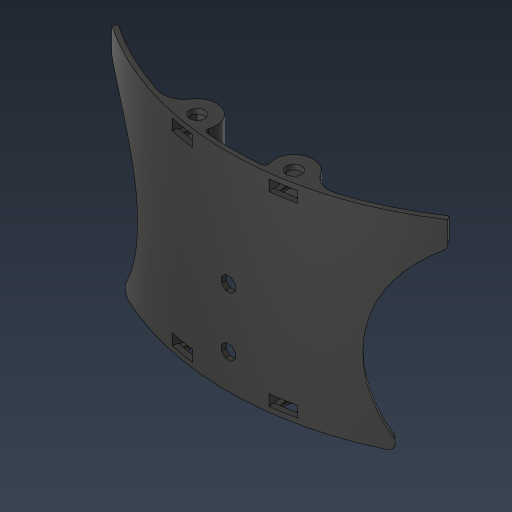
# Autodesk Inventor part: Verbindungsstrebe Hinten
Saved by Autodesk Inventor 2023.1 (Build 271208000, 208)
## iProperties
Part Number: Verbindungsstrebe Hinten
Material: PC/ABS-Kunststoff
Document SubType Name: Modeling
Designer: rYan
Density: 0.357273 g/cm^3
Appearance: Glatt - Schwarz
Mass: 6.26904 g
Surface Area: 111.071 cm^2
Volume: 17.5469 cm^3
Author: rYan
Autodesk Inventor part; units mm, degrees
sketch "Skizze1" plane through (0, 0, 0) normal (0, 0, 1) x (1, 0, 0)
  circle A0 centre (-14, -82) radius 2.5 construction
  line L0 (0, 18.1271) -> (0, -108.7625) projected
  arc A1 (-48.6498, -72.1263) -> (0, -87) centre (0, 0) ccw
  arc A2 (-47.8949, -71.0071) -> (0, -85.65) centre (0, 0) ccw
  line L1 (0, 0) -> (-48.6498, -72.1263)
  arc A3 (-8.7476, -83.9422) -> (-18.7856, -79.0917) centre (-14, -82) ccw
  arc A4 (-25.7143, -81.6988) -> (-18.7856, -79.0917) centre (-23.913, -75.9756) ccw
  arc A5 (-8.7476, -83.9422) -> (-7.9019, -85.2847) centre (-7.8096, -84.289) ccw
  dimension "d0" = 82
  dimension "d1" = 14
  dimension "d2" = 5
  dimension "d3" = 174
  dimension "d5" = 1.35
  dimension "d6" = 34
  dimension "d7" = 5.6
  dimension "d8" = 6
  dimension "d9" = 1
  constraints: 12 point on circle, 6 centre point, 4 coincident, 4 tangent, 3 point on line, 2 end point
  measures "d0" vertical distance of A0.centre point (0, 0)
  measures "d1" distance from line of L0 A0.centre
  measures "d2" diameter of A0
  measures "d3" diameter of A1
  measures "d5" radial gap between concentric circles of A1 A2
  measures "d6" angle of L0 L1
  measures "d7" radius of A3
  measures "d8" radius of A4
  measures "d9" radius of A5
extrude "Extrusion1" add sketch "Skizze1" against normal blind 60 contours L0 A1 L1 A2 | A2 A4 A3 A5
hole "Bohrung1" at (-14, -82, 0) direction (0, 0, -1) diameter 4.4 depth 6
ref_plane "Arbeitsebene1" through (0, 0, -1.48) normal (0, 0, 1) x (1, 0, 0)
sketch "Skizze2" plane through (0, 0, -1.48) normal (0, 0, 1) x (1, 0, 0)
  circle A0 centre (-14, -82) radius 2.2 construction
  line L0 (-17.1315, -78.951) -> (-13.2331, -77.5081)
  line L1 (-13.2331, -77.5081) -> (-10.0342, -80.1628)
  line L2 (-10.0342, -80.1628) -> (-10.7338, -84.2604)
  line L3 (-10.7338, -84.2604) -> (-14.6323, -85.7033)
  line L4 (-14.6323, -85.7033) -> (-17.8311, -83.0487)
  line L5 (-17.8311, -83.0487) -> (-17.1315, -78.951)
  line L6 (-14, -82) -> (0, 0) construction
  line L7 (-17.8311, -83.0487) -> (-18.6726, -87.9773)
  line L8 (-18.6726, -87.9773) -> (-11.5753, -89.1891)
  line L9 (-11.5753, -89.1891) -> (-10.7338, -84.2604)
  point P0 (-13.9327, -81.6057)
  dimension "d51" = 7.2
  dimension "d52" = 0.4
  dimension "d53" = 5
  constraints: 20 end point, 2 collinear, 1 perpendicular, 1 point on line, 14 other
  measures "d51" distance between parallel lines of L2 L5
  measures "d52" distance of L6.start point (-13.933, -81.606)
  measures "d53" distance of L4.end L7.end
extrude "Extrusion2" cut sketch "Skizze2" against normal blind 3.2
ref_plane "Arbeitsebene2" through (0, 0, 0) normal (0.7071068, 0.7071068, 0) x (0, 0, 1)
sketch "Skizze3" plane through (0, 0, 0) normal (0.7071068, 0.7071068, 0) x (0, 0, 1)
  circle A0 centre (-37, 0) radius 34
  line L0 (-85.2, 0) -> (14.2, 0) construction
  point P0 (0, 0)
  dimension "d25" = 37
  dimension "d26" = 68
  constraints: 1 centre point, 1 point on line
  measures "d25" distance of A0.centre point (0, 0)
  measures "d26" diameter of A0
extrude "Extrusion3" cut sketch "Skizze3" against normal through all
ref_plane "Arbeitsebene3" through (0, 0, -30) normal (0, 0, 1) x (1, 0, 0)
mirror "Spiegeln2" about plane through (0, 0, -30) normal (0, 0, 1) of "Bohrung1", "Extrusion2"
ref_plane "Arbeitsebene4" through (0, 0, 0) normal (0.9986295, -0.052336, 0) x (0, 0, 1)
sketch "Skizze4" plane through (0, 0, 0) normal (0.9986295, -0.052336, 0) x (0, 0, 1)
  line L0 (-60, 85.65) -> (0, 85.65) projected
  line L1 (0, 87) -> (-60, 87) projected
  line L2 (-43, 87) -> (-43, 85.65)
  line L3 (-52, 87) -> (-52, 85.65)
  line L4 (-72.0021, 0) -> (12.0003, 0) projected
  point P0 (0, 0)
  dimension "d31" = 9
  dimension "d32" = 8
  constraints: 4 end point, 4 point on line, 2 perpendicular
  measures "d31" distance between parallel lines of L3 L2
  measures "d32" distance from line of L1.end L3
revolve "Umdrehung1" [suppressed]
fillet "Rundung1" radius 2 2 edges at (-48.2728, -71.5673, -7.2564) (-40.7105, -76.1224, -60)
sketch "Skizze5" plane through (0, 0, -4.68) normal (0, 0, 1) x (1, 0, 0)
  circle A0 centre (-14, -82) radius 2.2 projected
  line L0 (-10.8216, -84.7745) -> (-17.9189, -83.5628)
  line L1 (-10.0811, -80.4372) -> (-17.1784, -79.2255)
  line L2 (-14, -82) -> (0, 0) construction
  arc A1 (-18.1779, -85.0797) -> (-11.0806, -86.2915) centre (0, 0) ccw projected
  line L3 (-10.0342, -80.1628) -> (-11.0806, -86.2915) projected
  line L4 (-13.2331, -77.5081) -> (-10.0342, -80.1628) projected
  line L5 (-17.1315, -78.951) -> (-13.2331, -77.5081) projected
  line L6 (-18.1779, -85.0797) -> (-17.1315, -78.951) projected
  line L7 (-12.2016, -84.5389) -> (-11.4611, -80.2016)
  line L8 (-16.5389, -83.7984) -> (-15.7984, -79.4611)
  point P0 (-13.6297, -79.8314)
  point P1 (-14.3703, -84.1686)
  point P2 (-16.1686, -81.6297)
  point P3 (-11.8314, -82.3703)
  constraints: 10 end point, 8 point on line, 4 perpendicular, 4 tangent, 1 coincident
extrude "Extrusion4" cut sketch "Skizze5" against normal blind 0.3 contours A0 L1 L7 | A0 L8 L1 | L7 L0 A0 | L7 L1 L3 L0 | A0 L0 L8 | L8 L0 L6 L1
extrude "Extrusion7" cut sketch "Skizze5" against normal blind 0.6 contours A0 L1 L7 | A0 L8 L1 | L7 L0 A0 | A0 L0 L8
sketch "Skizze6" plane through (-11.0806, -86.2915, -58.52) normal (0, 0, 1) x (0.9857364, -0.1682965, 0)
  circle A0 centre (-3.6, 3.7389) radius 2.2 projected
  line L0 (0, 1.5389) -> (-7.2, 1.5389)
  line L1 (0, 5.9389) -> (-7.2, 5.9389)
  line L2 (-3.6, 3.7389) -> (-3.6, 86.9255) construction
  arc A1 (-7.2, 0) -> (0, 0) centre (-3.6, 86.9255) ccw projected
  line L3 (0, 0) -> (0, 6.2174) projected
  line L4 (0, 6.2174) -> (-3.6, 8.2959) projected
  line L5 (-3.6, 8.2959) -> (-7.2, 6.2174) projected
  line L6 (-7.2, 6.2174) -> (-7.2, 0) projected
  line L7 (-1.4, 1.5389) -> (-1.4, 5.9389)
  line L8 (-5.8, 1.5389) -> (-5.8, 5.9389)
  point P0 (-3.6, 5.9389)
  point P1 (-3.6, 1.5389)
  point P2 (-5.8, 3.7389)
  point P3 (-1.4, 3.7389)
  constraints: 10 end point, 8 point on line, 4 perpendicular, 4 tangent, 1 coincident, 1 horizontal
extrude "Extrusion5" cut sketch "Skizze6" against normal blind 0.3 contours L7 L0 A0 | L7 L1 L3 L0 | A0 L1 L7 | A0 L8 L1 | L0 L8 A0 | L8 L0 L6 L1
extrude "Extrusion8" cut sketch "Skizze6" against normal blind 0.6 contours L7 L0 A0 | A0 L1 L7 | A0 L8 L1 | L0 L8 A0
mirror "Spiegeln1" about plane through (0, 0, 0) normal (1, 0, 0) of "Extrusion1", "Bohrung1", "Extrusion2", "Extrusion3", "Spiegeln2", "Rundung1", "Extrusion4", "Extrusion5", "Extrusion7", "Extrusion8"
sketch "Skizze7" plane through (0, 0, 0) normal (0, 1, 0) x (-1, 0, 0)
  line L0 (0, -72.0019) -> (0, 12.0003) construction
  line L1 (0.8284, -52) -> (-0.8284, -52)
  line L2 (-0.8284, -52) -> (-2, -50.8284)
  line L3 (-2, -50.8284) -> (-2, -49.1716)
  line L4 (-2, -49.1716) -> (-0.8284, -48)
  line L5 (-0.8284, -48) -> (0.8284, -48)
  line L6 (0.8284, -48) -> (2, -49.1716)
  line L7 (2, -49.1716) -> (2, -50.8284)
  line L8 (2, -50.8284) -> (0.8284, -52)
  line L9 (0.8284, -35) -> (-0.8284, -35)
  line L10 (-0.8284, -35) -> (-2, -33.8284)
  line L11 (-2, -33.8284) -> (-2, -32.1716)
  line L12 (-2, -32.1716) -> (-0.8284, -31)
  line L13 (-0.8284, -31) -> (0.8284, -31)
  line L14 (0.8284, -31) -> (2, -32.1716)
  line L15 (2, -32.1716) -> (2, -33.8284)
  line L16 (2, -33.8284) -> (0.8284, -35)
  line L17 (7.9019, -60) -> (-7.9019, -60) projected
  point P0 (0, 0)
  point P1 (0, -50)
  point P2 (0, -33)
  dimension "d41" = 4
  dimension "d43" = 50
  dimension "d44" = 10
  dimension "d45" = 17
  constraints: 32 end point, 2 horizontal, 2 point on line, 1 collinear, 34 other
  measures "d41" distance between parallel lines of L7 L3
  measures "d43" distance of point (0, -50) point (0, 0)
  measures "d44" distance from line of L17 point (0, -50)
  measures "d45" distance of point (0, -50) point (0, -33)
extrude "Extrusion6" cut sketch "Skizze7" against normal through all
